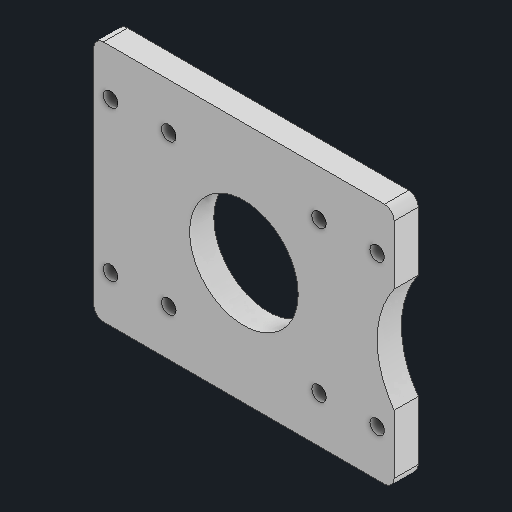
# Autodesk Inventor part: motor_cover_final
Saved by Autodesk Inventor 2024.2 (Build 282272000, 272)
## iProperties
Created: 2024-03-21
Part Number: motor_cover_final
Material: Generic
Document SubType Name: Modeling
Designer: seifs
Density: 1 g/cm^3
Appearance: Default
Author: seifs
Autodesk Inventor part; units mm, degrees
ref_plane "YZ Plane" through (0, 0, 0) normal (1, 0, 0) x (0, 1, 0)
ref_plane "XZ Plane" through (0, 0, 0) normal (0, 1, 0) x (-1, 0, 0)
ref_plane "XY Plane" through (0, 0, 0) normal (0, 0, 1) x (1, 0, 0)
sketch "Sketch1" plane through (0, 0, 0) normal (0, 0, 1) x (1, 0, 0)
  arc A0 (-15, 10.8282) -> (-15, -10.8282) centre (0, 0) ccw projected
  line L0 (-15, -23) -> (-15, -10.8282) projected
  line L1 (-15, 10.8282) -> (-15, 23) projected
  line L2 (-17, 25) -> (-75, 25) projected
  arc A1 (-15, 23) -> (-17, 25) centre (-17, 23) ccw projected
  arc A2 (-75, 25) -> (-77, 23) centre (-75, 23) ccw projected
  line L3 (-77, 23) -> (-77, -23) projected
  arc A3 (-77, -23) -> (-75, -25) centre (-75, -23) ccw projected
  line L4 (-75, -25) -> (-17, -25) projected
  arc A4 (-17, -25) -> (-15, -23) centre (-17, -23) ccw projected
  circle A5 centre (-18.5, -15.5) radius 1.5 projected
  circle A6 centre (-18.5, 15.5) radius 1.5 projected
  circle A7 centre (-73.5, 15.5) radius 1.5 projected
  circle A8 centre (-73.5, -15.5) radius 1.5 projected
  circle A9 centre (-60.15, -16.85) radius 1.5 construction
  circle A10 centre (-29.15, -16.85) radius 1.5 construction
  circle A11 centre (-29.15, 14.15) radius 1.5 construction
  circle A12 centre (-60.15, 14.15) radius 1.5 construction
  circle A13 centre (-29.15, 14.15) radius 1.5 construction
  circle A14 centre (-44.65, -1.35) radius 11.2 construction
  circle A15 centre (-44.65, -1.35) radius 11.2 construction
  circle A16 centre (-18.5, -15.5) radius 1.5
  circle A17 centre (-18.5, 15.5) radius 1.5
  circle A18 centre (-73.5, 15.5) radius 1.5
  circle A19 centre (-73.5, -15.5) radius 1.5
  line L5 (-17, -25) -> (-75, -25)
  line L6 (-77, -23) -> (-77, 23)
  line L7 (-75, 25) -> (-17, 25)
  arc A20 (-15, 23) -> (-17, 25) centre (-17, 23) ccw
  arc A21 (-17, -25) -> (-15, -23) centre (-17, -23) ccw
  arc A22 (-77, -23) -> (-75, -25) centre (-75, -23) ccw
  arc A23 (-75, 25) -> (-77, 23) centre (-75, 23) ccw
  line L8 (-15, 23) -> (-15, 10.8282)
  line L9 (-15, -10.8282) -> (-15, -23)
  arc A24 (-15, 10.8282) -> (-15, -10.8282) centre (0, 0) ccw
  line L10 (-23, -25) -> (-69, -25) projected
  line L11 (-23, -25) -> (-69, -25) projected
  line L12 (-46, -23) -> (-46, 0) construction
  circle A25 centre (-46, 0) radius 11.2
  line L13 (-46, 0) -> (-46, 15.5) construction
  line L14 (-46, 15.5) -> (-30.5, 15.5) construction
  line L15 (-46, 15.5) -> (-61.5, 15.5) construction
  circle A26 centre (-30.5, 15.5) radius 1.5
  circle A27 centre (-61.5, 15.5) radius 1.5
  line L16 (-46, 0) -> (-46, -15.5) construction
  line L17 (-46, -15.5) -> (-61.5, -15.5) construction
  line L18 (-46, -15.5) -> (-30.5, -15.5) construction
  circle A28 centre (-30.5, -15.5) radius 1.5
  circle A29 centre (-61.5, -15.5) radius 1.5
  point P0 (0, 0)
  dimension "d0" = 2
  dimension "d1" = 22.4
  dimension "d2" = 15.5
  dimension "d3" = 15.5
  dimension "d4" = 15.5
  dimension "d5" = 3
  dimension "d6" = 3
  dimension "d7" = 15.5
  dimension "d8" = 15.5
  dimension "d9" = 15.5
  dimension "d10" = 3
  dimension "d11" = 3
  constraints: 24 end point, 14 centre point, 12 point on circle, 10 tangent, 9 coincident, 7 equal radius, 4 horizontal, 3 parallel, 3 perpendicular, 2 point on line
  measures "d0" radius of A20
  measures "d1" diameter of A25
  measures "d2" distance of L13.start L13.end
  measures "d3" distance of L13.end L14.end
  measures "d4" distance of L13.end L15.end
  measures "d5" diameter of A26
  measures "d6" diameter of A27
  measures "d7" distance of L13.start L16.end
  measures "d8" distance of L16.end L17.end
  measures "d9" distance of L16.end L18.end
  measures "d10" diameter of A28
  measures "d11" diameter of A29
extrude "Extrusion1" add sketch "Sketch1" along normal blind 5
body "Solid1"
